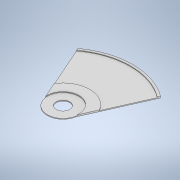
# Autodesk Inventor part: shutter
Saved by Autodesk Inventor 2021 (Build 250183000, 183)
## iProperties
Created: 2024-02-08
Part Number: shutter
Material: Generic
Document SubType Name: Modeling
Designer: Sebastián
Density: 1 g/cm^3
Appearance: Default
Author: Sebastián
Autodesk Inventor part; units mm, degrees
ref_plane "YZ Plane" through (0, 0, 0) normal (1, 0, 0) x (0, 1, 0)
ref_plane "XZ Plane" through (0, 0, 0) normal (0, 1, 0) x (-1, 0, 0)
ref_plane "XY Plane" through (0, 0, 0) normal (0, 0, 1) x (1, 0, 0)
sketch "Sketch1" plane through (0, 0, 0) normal (0, 1, 0) x (-1, 0, 0)
  circle A0 centre (0, 0) radius 74.5 construction
  circle A1 centre (0, 30) radius 44.5 construction
  circle A2 centre (0, 30) radius 4.3
  circle A3 centre (0, 30) radius 10 construction
  arc A4 (9.8601, 31.6667) -> (-9.8601, 31.6667) centre (0, 30) ccw construction
  line L0 (0, -104.3) -> (0, 104.3) construction
  arc A5 (9.8601, 31.6667) -> (-9.8601, 31.6667) centre (0, 30) ccw
  line L1 (9.8601, 31.6667) -> (26.4003, -5.8228)
  arc A6 (-26.4003, -5.8228) -> (26.4003, -5.8228) centre (0, 30) ccw
  line L2 (-9.8601, 31.6667) -> (-26.4003, -5.8228)
  dimension "d5" = 20
  dimension "d0" = 149
  dimension "d3" = 30
  dimension "d4" = 8.6
  constraints: 9 point on circle, 6 centre point, 6 coincident, 4 end point, 1 concentric, 1 point on line, 1 symmetric about line, 1 tangent, 3 other
  measures "d0" diameter of A0
  measures "d3" distance of A1.centre point (0, 0)
  measures "d4" diameter of A2
extrude "Extrusion1" add sketch "Sketch1" along normal blind 1
sketch "Sketch2" plane through (0, 1, 0) normal (0, 1, 0) x (1, 0, 0)
  circle A0 centre (0, -30) radius 4.3 construction
  circle A1 centre (0, -30) radius 10.2
  point P0 (0, 0)
  dimension "d8" = 20.4
  constraints: 1 centre point, 1 coincident
  measures "d8" diameter of A1
extrude "Extrusion2" cut sketch "Sketch2" against normal blind 0.5
sketch "Sketch3" plane through (0, 1, 0) normal (0, 1, 0) x (1, 0, 0)
  circle A0 centre (0, -30) radius 4.3 construction
  line L0 (9.8601, -31.6667) -> (26.4003, 5.8228) construction
  circle A1 centre (0, -30) radius 4.3 construction
  arc A2 (25.9919, 4.2553) -> (-25.7794, 4.4155) centre (0, -30) ccw
  arc A3 (14.5062, -21.136) -> (-14.5062, -21.136) centre (0, -30) ccw
  line L1 (14.5062, -21.136) -> (25.9919, 4.2553)
  line L2 (-26.4003, 5.8228) -> (-9.8601, -31.6667) projected
  line L3 (-14.5062, -21.136) -> (-25.7794, 4.4155)
  point P0 (0, 0)
  point P1 (-25.7794, 4.4155)
  dimension "d12" = 43
  dimension "d13" = 17
  constraints: 4 end point, 4 point on circle, 2 centre point, 2 coincident, 2 point on line, 1 collinear
  measures "d12" radius of A2
  measures "d13" radius of A3
extrude "Extrusion3" cut sketch "Sketch3" against normal blind 0.4
body "Solid1"
